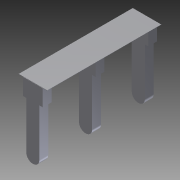
# Autodesk Inventor part: M2T1SW03trmnls
Saved by Autodesk Inventor 2011 SP1 (Build 150282100, 282)
## iProperties
Created: 2013-12-24
Part Number: M2T1SW03trmnls
Catalog Web Link: www.cadenas.de
Description: M2T Series - Process Sealed Miniature Toggles - Terminals-
Vendor: NKKSWITCHES
Document SubType Name: Modeling
Designer: PARTuser1
Manufacturer: NKKSWITCHES
Density: 1 g/cm^3
Category: PARTsolutions
Company: NKKSWITCHES
Title: M2T1SW03trmnls
Author: Cadenas PARTsolutions
PSOL_IDENT_0: {$CADENAS_DATA\23d-libs\nkkswitches\toggle\m2t\parts\m2t_terminals.prj},240 {VTYP=3D},{NB=M2T1SW03tr
PSOL_IDENT_1: mnls},{LINA=M2T1SW03trmnls},{NN=M2T Series - Process Sealed Miniature Toggles - Terminals},{DATE=02.
PSOL_IDENT_2: 04.2013 12:03:38},{GEOMDATE=02.04.2013 14:03:00},{VERSION=},{LINEID=10},{LINESUBID=-1},{WBVAR=PLS,AC
PSOL_IDENT_3: TU,CMR,TRMNLS}  {NB=M2T1SW03trmnls},{LINA=M2T1SW03trmnls},{KT=DUMMY},{PN=M2T1SW03},{SRS=M2T},{PLS=1}
PSOL_IDENT_4: ,{ACTU=S},{CMR=W},{TRMNLS=03},{ALG= '03','03 - Straight','05','05 - .390\" (9.9mm) Extended PC','06'
PSOL_IDENT_5: ,'06 - .728\" (18.5mm) Extended PC','07','07 - .945\" (24.0mm) Extended PC' },{A=0.232},{CMRALG=0.75
PSOL_IDENT_6: ,0.75,0.75,0.00}
CNS_NN: M2T Series - Process Sealed Miniature Toggles - Terminals
CNS_NB: M2T1SW03trmnls
CNS_NBSYN: $PN.trmnls
CNS_LINA: M2T1SW03trmnls
CNS_PN: M2T1SW03
CNS_SRS: M2T
CNS_PLS: 1 - SPDT
CNS_ACTU: S - .500" (12.7mm) Bat Lever
CNS_CMR: W - Silver; Rated 6A @ 125V AC & 3A @ 250V AC
CNS_TRMNLS: 03 - Straight
CNS_ALG: '03','03 - Straight','05','05 - .390" (9.9mm) Extended PC','06','06 - .728" (18.5mm) Extended PC','07','07 - .945" (24.0mm) Extended PC'
CNS_A: 0.232
CNS_CMRALG: 0.75,0.75,0.75,0.00
SUPPLIER: NKKSWITCHES
ARTICLENO: M2T1SW03trmnls
BOMINFO: M2T1SW03trmnls
CREATOR: CADENAS GmbH
Autodesk Inventor part; units mm, degrees
sketch "Sketch_44" plane through (0, 0.254, 0) normal (0, 1, 0) x (1, 0, 0)
  line L0 (-1.27, -5.08) -> (1.27, -5.08)
  line L1 (1.27, -5.08) -> (1.27, 5.08)
  line L2 (1.27, 5.08) -> (-1.27, 5.08)
  line L3 (-1.27, 5.08) -> (-1.27, -5.08)
  constraints: 8 end point
extrude "Extrusion1" add sketch "Sketch_44" along normal blind 0.0254
sketch "Sketch_2" plane through (0, 0, 0) normal (0, 0, 1) x (1, 0, 0)
  line L0 (-0.889, 0.254) -> (-0.889, -1.2192)
  line L1 (-0.889, -1.2192) -> (-0.5842, -1.2192)
  line L2 (-0.5842, -1.2192) -> (-0.5842, -5.4356)
  arc A0 (-0.5842, -5.4356) -> (0.5842, -5.4356) centre (0, -5.4356) ccw
  line L3 (0.5842, -5.4356) -> (0.5842, -1.2192)
  line L4 (0.5842, -1.2192) -> (0.889, -1.2192)
  line L5 (0.889, -1.2192) -> (0.889, 0.254)
  line L6 (0.889, 0.254) -> (-0.889, 0.254)
  constraints: 14 end point, 2 point on circle, 1 centre point
extrude "Extrusion2" add sketch "Sketch_2" along normal mid plane 0.7874
sketch "Sketch_3" plane through (0, 0, 4.699) normal (0, 0, 1) x (1, 0, 0)
  line L0 (-0.889, 0.254) -> (-0.889, -1.2192)
  line L1 (-0.889, -1.2192) -> (-0.5842, -1.2192)
  line L2 (-0.5842, -1.2192) -> (-0.5842, -5.4356)
  arc A0 (-0.5842, -5.4356) -> (0.5842, -5.4356) centre (0, -5.4356) ccw
  line L3 (0.5842, -5.4356) -> (0.5842, -1.2192)
  line L4 (0.5842, -1.2192) -> (0.889, -1.2192)
  line L5 (0.889, -1.2192) -> (0.889, 0.254)
  line L6 (0.889, 0.254) -> (-0.889, 0.254)
  constraints: 14 end point, 2 point on circle, 1 centre point
extrude "Extrusion3" add sketch "Sketch_3" along normal mid plane 0.7874
sketch "Sketch_4" plane through (0, 0, -4.699) normal (0, 0, 1) x (1, 0, 0)
  line L0 (-0.889, 0.254) -> (-0.889, -1.2192)
  line L1 (-0.889, -1.2192) -> (-0.5842, -1.2192)
  line L2 (-0.5842, -1.2192) -> (-0.5842, -5.4356)
  arc A0 (-0.5842, -5.4356) -> (0.5842, -5.4356) centre (0, -5.4356) ccw
  line L3 (0.5842, -5.4356) -> (0.5842, -1.2192)
  line L4 (0.5842, -1.2192) -> (0.889, -1.2192)
  line L5 (0.889, -1.2192) -> (0.889, 0.254)
  line L6 (0.889, 0.254) -> (-0.889, 0.254)
  constraints: 14 end point, 2 point on circle, 1 centre point
extrude "Extrusion4" add sketch "Sketch_4" along normal mid plane 0.7874
ref_plane "body_right_vert_XY" through (0, 0, 0) normal (0, 0, -1) x (1, 0, 0)
ref_plane "body_right_vert_YZ" through (0, 0, 0) normal (1, 0, 0) x (0, -1, 0)
ref_plane "body_right_vert_ZX" through (0, 0, 0) normal (0, -1, 0) x (0, 0, -1)
ref_plane "body_straight_XY" through (0, 0, 0) normal (0, -1, 0) x (1, 0, 0)
ref_plane "body_straight_YZ" through (0, 0, 0) normal (1, 0, 0) x (0, 0, 1)
ref_plane "body_straight_ZX" through (0, 0, 0) normal (0, 0, 1) x (0, -1, 0)
body "Solid1"
